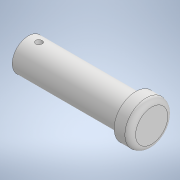
# Autodesk Inventor part: Lift.03.00.00.03
Saved by Autodesk Inventor 2021 (Build 250183000, 183)
## iProperties
Created: 2020-09-20
Part Number: Lift.03.00.00.03
Material: Типовые
Document SubType Name: Modeling
Designer: Kostya
Density: 1 g/cm^3
Appearance: По умолчанию
Author: Kostya
Autodesk Inventor part; units mm, degrees
ref_plane "YZ Plane" through (0, 0, 0) normal (1, 0, 0) x (0, 1, 0)
ref_plane "XZ Plane" through (0, 0, 0) normal (0, 1, 0) x (-1, 0, 0)
ref_plane "XY Plane" through (0, 0, 0) normal (0, 0, 1) x (1, 0, 0)
sketch "Эскиз1" plane through (0, 0, 0) normal (0, 0, 1) x (1, 0, 0)
  line L0 (0, 0) -> (-282.435, 0)
  line L1 (0, 0) -> (0, 30)
  line L2 (-10, 40) -> (-30, 40)
  line L3 (-30, 40) -> (-30, 30)
  line L4 (-30, 30) -> (-230, 30)
  line L5 (-230, 30) -> (-230, 0)
  arc A0 (0, 30) -> (-10, 40) centre (-10, 30) ccw
  point P0 (0, 40)
  dimension "d0" = 230
  dimension "d1" = 80
  dimension "d2" = 60
  dimension "d3" = 30
  dimension "d4" = 10
  constraints: 12 end point, 4 perpendicular, 3 point on line, 2 point on circle, 2 tangent, 1 centre point, 1 horizontal, 1 vertical
  measures "d0" distance between parallel lines of L5 L1
  measures "d1" diameter of L2 L0
  measures "d2" diameter of L4 L0
  measures "d3" distance of point (0, 40) L2.end
  measures "d4" radius of A0
revolve "Вращение1" add sketch "Эскиз1" angle 360 about axis through (0, 0, 0) along (-1, 0, 0)
sketch "Эскиз2" plane through (0, 0, 0) normal (0, 1, 0) x (-1, 0, 0)
  line L0 (230, 30) -> (230, -30) projected
  line L1 (30, 30) -> (30, -30) projected
  circle A0 centre (210, 0) radius 6
  point P0 (0, 0)
  point P1 (230, 0)
  dimension "d6" = 12
  dimension "d7" = 20
  constraints: 1 centre point, 1 horizontal alignment, 1 midpoint
  measures "d6" diameter of A0
  measures "d7" distance from line of A0.centre L0
extrude "Выдавливание1" cut sketch "Эскиз2" against normal through all both and the other way through all
